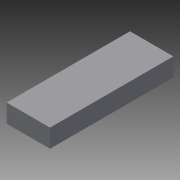
# Autodesk Inventor part: Catapult Base
Saved by Autodesk Inventor 2015 (Build 190159000, 159)
## iProperties
Created: 2016-02-06
Part Number: Catapult Base
Material: Generic
Document SubType Name: Modeling
Designer: sethbattis
Density: 1 g/cm^3
Appearance: Default
Author: sethbattis
Autodesk Inventor part; units mm, degrees
ref_plane "YZ Plane" through (0, 0, 0) normal (1, 0, 0) x (0, 1, 0)
ref_plane "XZ Plane" through (0, 0, 0) normal (0, 1, 0) x (-1, 0, 0)
ref_plane "XY Plane" through (0, 0, 0) normal (0, 0, 1) x (1, 0, 0)
sketch "Sketch1" plane through (0, 0, 0) normal (0, 1, 0) x (-1, 0, 0)
  line L0 (120.65, 342.9) -> (-120.65, 342.9)
  line L1 (-120.65, 342.9) -> (-120.65, -342.9)
  line L2 (-120.65, -342.9) -> (120.65, -342.9)
  line L3 (120.65, -342.9) -> (120.65, 342.9)
  line L4 (0, -480.06) -> (0, 480.06) construction
  line L5 (168.91, 0) -> (-168.91, 0) construction
  point P0 (0, 0)
  dimension "d0" = 241.3
  dimension "d1" = 685.8
  constraints: 8 end point, 2 parallel, 1 horizontal, 1 perpendicular, 2 other
  measures "d0" distance of L2.end L1.end
  measures "d1" distance of L1.end L0.end
extrude "Extrusion1" add sketch "Sketch1" along normal blind 101.6
body "Solid1"
